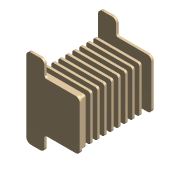
# Autodesk Inventor part: bobbin-2
Saved by Autodesk Inventor 2015 (Build 190159000, 159)
## iProperties
Created: 2014-10-07
Part Number: bobbin-2
Material: Polyethylene, Low Density
Document SubType Name: Modeling
Designer: Adam
Density: 0.894 g/cm^3
Appearance: Smooth - Off-White
Author: Adam
Autodesk Inventor part; units mm, degrees
ref_plane "Work Plane1" through (0, 0, 0.5) normal (0, 0, 1) x (1, 0, 0)
sketch "Sketch1" plane through (0, 0, 0.5) normal (0, 0, 1) x (1, 0, 0)
  line L0 (0, -12.7) -> (9.53, -12.7) construction
  line L1 (9.53, -4.565) -> (9.53, -12.7) construction
  line L2 (0, -4.565) -> (9.53, -4.565) construction
  line L3 (0, -4.565) -> (0, -12.7) construction
  line L4 (9.53, -22.23) -> (0, -22.23) construction
  line L5 (0, -22.23) -> (0, -30.365) construction
  line L6 (0, -30.365) -> (9.53, -30.365) construction
  line L7 (9.53, -22.23) -> (9.53, -30.365) construction
  line L8 (0, -22.23) -> (0, -12.7) construction
  line L9 (9.53, -12.7) -> (9.53, -22.23) construction
  line L10 (-0.5, -22.73) -> (10.03, -22.73)
  line L11 (10.03, -22.73) -> (10.03, -12.2)
  line L12 (10.03, -12.2) -> (-0.5, -12.2)
  line L13 (-0.5, -12.2) -> (-0.5, -22.73)
  line L14 (-0.5, -29.865) -> (10.03, -29.865)
  line L15 (10.03, -29.865) -> (10.03, -22.73)
  line L16 (10.03, -22.73) -> (-0.5, -22.73)
  line L17 (-0.5, -22.73) -> (-0.5, -29.865)
  line L18 (-0.5, -12.2) -> (10.03, -12.2)
  line L19 (10.03, -12.2) -> (10.03, -5.065)
  line L20 (10.03, -5.065) -> (-0.5, -5.065)
  line L21 (-0.5, -5.065) -> (-0.5, -12.2)
  line L22 (-0.5, -29.865) -> (-7.635, -29.865)
  line L23 (-7.635, -29.865) -> (-7.635, -5.065)
  line L24 (-7.635, -5.065) -> (-0.5, -5.065)
  line L25 (-0.5, -5.065) -> (-0.5, -29.865)
  line L26 (10.03, -29.865) -> (17.165, -29.865)
  line L27 (17.165, -29.865) -> (17.165, -5.065)
  line L28 (17.165, -5.065) -> (10.03, -5.065)
  line L29 (10.03, -5.065) -> (10.03, -29.865)
  point P0 (0, 0)
  dimension "d1" = 0.5
  dimension "d2" = 0.5
  dimension "d3" = 0.5
  dimension "d4" = 0.5
  dimension "d5" = 0.5
  dimension "d6" = 0.5
  dimension "d7" = 7.135
  dimension "d8" = 7.135
  dimension "d9" = 7.135
  constraints: 44 end point, 11 parallel, 5 horizontal, 5 perpendicular, 4 collinear, 1 vertical
  measures "d1" distance between parallel lines of L0 L12
  measures "d2" distance between parallel lines of L4 L10
  measures "d3" distance between parallel lines of L8 L13
  measures "d4" distance between parallel lines of L11 L9
  measures "d5" distance between parallel lines of L6 L14
  measures "d6" distance between parallel lines of L20 L2
  measures "d7" distance of L16.end L14.start
  measures "d8" distance between parallel lines of L23 L25
  measures "d9" distance between parallel lines of L11 L27
extrude "Extrusion1" add sketch "Sketch1" along normal blind 1.2 contours L17 L22 L23 L24 L21 L13 | L10 L15 L14 L17 | L11 L19 L28 L27 L26 L15 | L21 L20 L19 L12
sketch "Sketch2" plane through (0, 0, 1.7) normal (0, 0, 1) x (1, 0, 0)
  line L0 (-7.635, -29.865) -> (17.165, -29.865) construction
  line L1 (17.165, -29.865) -> (17.165, -5.065) construction
  line L2 (17.165, -5.065) -> (-7.635, -5.065) construction
  line L3 (-7.635, -5.065) -> (-7.635, -29.865) construction
  line L4 (-0.5, -22.73) -> (-0.5, -12.2) projected
  line L5 (-0.5, -12.2) -> (10.03, -12.2) projected
  line L6 (10.03, -12.2) -> (10.03, -22.73) projected
  line L7 (10.03, -22.73) -> (-0.5, -22.73) projected
  line L8 (-1.7, -23.93) -> (11.23, -23.93)
  line L9 (11.23, -23.93) -> (11.23, -11)
  line L10 (11.23, -11) -> (-1.7, -11)
  line L11 (-1.7, -11) -> (-1.7, -23.93)
  point P0 (0, 0)
  dimension "d12" = 1.2
  dimension "d13" = 1.2
  dimension "d14" = 1.2
  dimension "d15" = 1.2
  constraints: 8 end point, 2 parallel, 1 horizontal, 1 perpendicular
  measures "d12" distance between parallel lines of L4 L11
  measures "d13" distance between parallel lines of L8 L7
  measures "d14" distance between parallel lines of L10 L5
  measures "d15" distance between parallel lines of L6 L9
ref_plane "Work Plane2" through (0, -35.0828, 37.6) normal (0, 0, -1) x (1, 0, 0)
extrude "Extrusion2" add sketch "Sketch2" along normal up to surface (35.9 mm away)
sketch "Sketch3" plane through (-1.7, -23.93, 37.6) normal (0, 0, 1) x (1, 0, 0)
  line L0 (1.2, 11.73) -> (11.73, 11.73) construction
  line L1 (11.73, 11.73) -> (11.73, 1.2) construction
  line L2 (11.73, 1.2) -> (1.2, 1.2) construction
  line L3 (1.2, 1.2) -> (1.2, 11.73) construction
  line L4 (0, 12.93) -> (0, 0) construction
  line L5 (0, 0) -> (12.93, 0) construction
  line L6 (12.93, 0) -> (12.93, 12.93) construction
  line L7 (12.93, 12.93) -> (0, 12.93) construction
  line L8 (-5.935, -5.935) -> (18.865, -5.935)
  line L9 (18.865, -5.935) -> (18.865, 18.865)
  line L10 (18.865, 18.865) -> (-5.935, 18.865)
  line L11 (-5.935, 18.865) -> (-5.935, -5.935)
  line L12 (12.93, 0) -> (0, 0) construction
  line L13 (0, 0) -> (0, 12.93) construction
  line L14 (0, 12.93) -> (12.93, 12.93) construction
  line L15 (12.93, 12.93) -> (12.93, 0) construction
  line L16 (-5.935, -5.935) -> (18.865, -5.935) construction
  line L17 (18.865, -5.935) -> (18.865, 18.865) construction
  line L18 (18.865, 18.865) -> (-5.935, 18.865) construction
  line L19 (-5.935, 18.865) -> (-5.935, -5.935) construction
  line L20 (0, 0) -> (12.93, 0)
  line L21 (12.93, 0) -> (12.93, 12.93)
  line L22 (12.93, 12.93) -> (0, 12.93)
  line L23 (0, 12.93) -> (0, 0)
  point P0 (1.7, 23.93)
  constraints: 16 end point, 4 collinear, 4 parallel, 2 horizontal, 2 perpendicular
extrude "Extrusion3" add sketch "Sketch3" against normal blind 1.2
ref_plane "Work Plane3" through (-1.7, -23.93, 34.9) normal (0, 0, -1) x (-1, 0, 0)
sketch "Sketch4" plane through (-1.7, -23.93, 34.9) normal (0, 0, -1) x (-1, 0, 0)
  line L0 (5, 17.93) -> (-17.93, 17.93)
  line L1 (-17.93, 17.93) -> (-17.93, -5)
  line L2 (-17.93, -5) -> (5, -5)
  line L3 (5, -5) -> (5, 17.93)
  line L4 (0, 0) -> (0, 12.93) projected
  line L5 (-12.93, 0) -> (0, 0) projected
  line L6 (-12.93, 12.93) -> (-12.93, 0) projected
  line L7 (0, 12.93) -> (-12.93, 12.93) projected
  point P0 (-1.7, 23.93)
  dimension "d21" = 5
  dimension "d22" = 5
  dimension "d23" = 5
  dimension "d24" = 5
  constraints: 8 end point, 2 parallel, 1 horizontal, 1 perpendicular
  measures "d21" distance between parallel lines of L2 L5
  measures "d22" distance between parallel lines of L6 L1
  measures "d23" distance between parallel lines of L7 L0
  measures "d24" distance between parallel lines of L4 L3
extrude "Extrusion4" add sketch "Sketch4" along normal blind 1.2
fillet "Fillet1" radius 1 4 edges at (-6.7, -28.93, 34.3) (-6.7, -6, 34.3) (16.23, -28.93, 34.3) (16.23, -6, 34.3)
pattern_linear "Rectangular Pattern1" count 9 spacing 3.5 along (0, 0, -1) of "Extrusion4", "Fillet1"
fillet "Fillet2" radius 2 8 edges at (-7.635, -29.865, 37) (17.165, -29.865, 37) (17.165, -5.065, 37) (-7.635, -5.065, 37) (-7.635, -5.065, 1.1) (-7.635, -29.865, 1.1) (17.165, -29.865, 1.1) (17.165, -5.065, 1.1)
fillet "Fillet2" radius 1.5 4 edges at (11.23, -11, 3.7) (11.23, -23.93, 3.7) (-1.7, -11, 3.7) (-1.7, -23.93, 3.7)
fillet "Fillet2" radius 1 4 edges at (-0.5, -12.2, 19.05) (-0.5, -22.73, 19.05) (10.03, -22.73, 19.05) (10.03, -12.2, 19.05)
sketch "Sketch5" plane through (-5.635, -29.865, 37.6) normal (0, 0, 1) x (1, 0, 0)
  arc A0 (0, 24.8) -> (-2, 22.8) centre (0, 22.8) ccw construction
  line L0 (-2, 22.8) -> (-2, 2) construction
  arc A1 (-2, 2) -> (0, 0) centre (0, 2) ccw construction
  line L1 (0, 0) -> (20.8, 0) construction
  arc A2 (20.8, 0) -> (22.8, 2) centre (20.8, 2) ccw construction
  line L2 (22.8, 2) -> (22.8, 22.8) construction
  arc A3 (22.8, 22.8) -> (20.8, 24.8) centre (20.8, 22.8) ccw construction
  line L3 (20.8, 24.8) -> (0, 24.8) construction
  line L4 (6.135, 17.665) -> (14.665, 17.665) construction
  line L5 (15.665, 16.665) -> (15.665, 8.135) construction
  line L6 (14.665, 7.135) -> (6.135, 7.135) construction
  line L7 (5.135, 8.135) -> (5.135, 16.665) construction
  arc A4 (0, 24.8) -> (-2, 22.8) centre (0, 22.8) ccw projected
  line L8 (0, 24.8) -> (20.8, 24.8) projected
  arc A5 (22.8, 22.8) -> (20.8, 24.8) centre (20.8, 22.8) ccw projected
  line L9 (22.8, 22.8) -> (22.8, 2) projected
  arc A6 (20.8, 0) -> (22.8, 2) centre (20.8, 2) ccw projected
  line L10 (20.8, 0) -> (0, 0) projected
  arc A7 (-2, 2) -> (0, 0) centre (0, 2) ccw projected
  line L11 (-2, 2) -> (-2, 22.8) projected
  line L12 (16.865, 17.365) -> (16.865, 7.435) projected
  line L13 (5.435, 18.865) -> (15.365, 18.865) projected
  line L14 (3.935, 7.435) -> (3.935, 17.365) projected
  line L15 (15.365, 5.935) -> (5.435, 5.935) projected
  line L16 (3.435, 4.435) -> (17.365, 4.435)
  line L17 (18.365, 5.435) -> (18.365, 19.365)
  line L18 (17.365, 20.365) -> (3.435, 20.365)
  line L19 (2.435, 19.365) -> (2.435, 5.435)
  arc A8 (2.435, 5.435) -> (3.435, 4.435) centre (3.435, 5.435) ccw
  arc A9 (17.365, 4.435) -> (18.365, 5.435) centre (17.365, 5.435) ccw
  arc A10 (18.365, 19.365) -> (17.365, 20.365) centre (17.365, 19.365) ccw
  arc A11 (3.435, 20.365) -> (2.435, 19.365) centre (3.435, 19.365) ccw
  arc A12 (15.665, 16.665) -> (14.665, 17.665) centre (14.665, 16.665) ccw projected
  arc A13 (14.665, 7.135) -> (15.665, 8.135) centre (14.665, 8.135) ccw projected
  arc A14 (5.135, 8.135) -> (6.135, 7.135) centre (6.135, 8.135) ccw projected
  arc A15 (6.135, 17.665) -> (5.135, 16.665) centre (6.135, 16.665) ccw projected
  arc A16 (15.365, 5.935) -> (16.865, 7.435) centre (15.365, 7.435) ccw projected
  arc A17 (16.865, 17.365) -> (15.365, 18.865) centre (15.365, 17.365) ccw projected
  arc A18 (5.435, 18.865) -> (3.935, 17.365) centre (5.435, 17.365) ccw projected
  arc A19 (3.935, 7.435) -> (5.435, 5.935) centre (5.435, 7.435) ccw projected
  point P0 (5.635, 29.865)
  dimension "d32" = 1.5
  dimension "d33" = 1.5
  dimension "d34" = 1.5
  dimension "d35" = 1.5
  dimension "d36" = 1
  constraints: 8 end point, 8 point on circle, 8 tangent, 4 centre point, 3 equal radius, 2 parallel, 1 horizontal, 1 perpendicular
  measures "d32" distance between parallel lines of L18 L13
  measures "d33" distance between parallel lines of L14 L19
  measures "d34" distance between parallel lines of L16 L15
  measures "d35" distance between parallel lines of L17 L12
  measures "d36" radius of A8
extrude "Extrusion5" add sketch "Sketch5" against normal up to surface (30.7 mm away) contours A8 L19 A11 L18 A10 L17 A9 L16
sketch "Sketch6" plane through (-6.7, -27.93, 10.4) normal (-1, 0, 0) x (0, 0, 1)
  line L0 (5.8, 20.93) -> (7, 20.93) construction
  line L1 (5.8, 0) -> (5.8, 20.93) construction
  line L2 (7, 0) -> (5.8, 0) construction
  line L3 (7, 0) -> (7, 20.93) construction
  line L4 (9.3, 20.93) -> (10.5, 20.93) construction
  line L5 (9.3, 0) -> (9.3, 20.93) construction
  line L6 (10.5, 0) -> (9.3, 0) construction
  line L7 (10.5, 0) -> (10.5, 20.93) construction
  line L8 (12.8, 20.93) -> (14, 20.93) construction
  line L9 (12.8, 0) -> (12.8, 20.93) construction
  line L10 (14, 0) -> (12.8, 0) construction
  line L11 (14, 0) -> (14, 20.93) construction
  line L12 (16.3, 20.93) -> (17.5, 20.93) construction
  line L13 (16.3, 0) -> (16.3, 20.93) construction
  line L14 (17.5, 0) -> (16.3, 0) construction
  line L15 (17.5, 0) -> (17.5, 20.93) construction
  line L16 (19.8, 20.93) -> (21, 20.93) construction
  line L17 (19.8, 0) -> (19.8, 20.93) construction
  line L18 (21, 0) -> (19.8, 0) construction
  line L19 (21, 0) -> (21, 20.93) construction
  line L20 (23.3, 20.93) -> (24.5, 20.93) construction
  line L21 (23.3, 0) -> (23.3, 20.93) construction
  line L22 (24.5, 0) -> (23.3, 0) construction
  line L23 (24.5, 0) -> (24.5, 20.93) construction
  line L24 (2.3, 20.93) -> (3.5, 20.93) construction
  line L25 (2.3, 0) -> (2.3, 20.93) construction
  line L26 (3.5, 0) -> (2.3, 0) construction
  line L27 (3.5, 0) -> (3.5, 20.93) construction
  line L28 (2.3, 0) -> (2.3, 20.93)
  line L29 (2.3, 11.965) -> (3.5, 11.965)
  line L30 (3.5, 11.965) -> (3.5, 8.965)
  line L31 (3.5, 8.965) -> (2.3, 8.965)
  line L32 (2.3, 8.965) -> (2.3, 11.965)
  line L33 (5.8, 0) -> (5.8, 20.93)
  line L34 (7, 3.5) -> (7, 17.43)
  line L35 (5.8, 11.965) -> (7, 11.965)
  line L36 (7, 11.965) -> (7, 8.965)
  line L37 (7, 8.965) -> (5.8, 8.965)
  line L38 (5.8, 8.965) -> (5.8, 11.965)
  line L39 (9.3, 17.43) -> (9.3, 3.5)
  line L40 (10.5, 0) -> (10.5, 20.93)
  line L41 (9.3, 11.965) -> (10.5, 11.965)
  line L42 (10.5, 11.965) -> (10.5, 8.965)
  line L43 (10.5, 8.965) -> (9.3, 8.965)
  line L44 (9.3, 8.965) -> (9.3, 11.965)
  line L45 (12.8, 17.43) -> (12.8, 3.5)
  line L46 (12.8, 11.965) -> (14, 11.965)
  line L47 (14, 11.965) -> (14, 8.965)
  line L48 (14, 8.965) -> (12.8, 8.965)
  line L49 (12.8, 8.965) -> (12.8, 11.965)
  line L50 (17.5, 17.43) -> (17.5, 3.5)
  line L51 (16.3, 11.965) -> (17.5, 11.965)
  line L52 (17.5, 11.965) -> (17.5, 8.965)
  line L53 (17.5, 8.965) -> (16.3, 8.965)
  line L54 (16.3, 8.965) -> (16.3, 11.965)
  line L55 (21, 17.43) -> (21, 3.5)
  line L56 (19.8, 11.965) -> (21, 11.965)
  line L57 (21, 11.965) -> (21, 8.965)
  line L58 (21, 8.965) -> (19.8, 8.965)
  line L59 (19.8, 8.965) -> (19.8, 11.965)
  line L60 (23.3, 11.965) -> (24.5, 11.965)
  line L61 (24.5, 11.965) -> (24.5, 8.965)
  line L62 (24.5, 8.965) -> (23.3, 8.965)
  line L63 (23.3, 8.965) -> (23.3, 11.965)
  line L64 (2.3, 10.465) -> (24.5, 10.465) construction
  line L65 (24.5, 20.93) -> (24.5, 0) construction
  line L66 (0, 3.5) -> (0, 17.43)
  line L67 (0, 8.965) -> (-1.2, 8.965)
  line L68 (-1.2, 8.965) -> (-1.2, 11.965)
  line L69 (-1.2, 11.965) -> (0, 11.965)
  line L70 (0, 11.965) -> (0, 8.965)
  line L71 (-1.2, 0) -> (-1.2, 20.93)
  line L72 (-3.5, 14.73) -> (-3.5, 6.2)
  line L73 (-4.7, 9.465) -> (-3.5, 9.465)
  line L74 (-3.5, 9.465) -> (-3.5, 11.465)
  line L75 (-3.5, 11.465) -> (-4.7, 11.465)
  line L76 (-4.7, 11.465) -> (-4.7, 9.465)
  line L77 (-4.7, 0) -> (-4.7, 20.93)
  point P0 (-10.4, 27.93)
extrude "Extrusion6" cut sketch "Sketch6" against normal up to surface (3.5 mm away) contours L28 L29 L30 L31 | L33 L35 L34 L37 | L41 L40 L43 L39 | L46 L47 L48 L45 | L50 L53 L54 L51 | L55 L58 L59 L56 | L67 L68 L69 L66 | L72 L73 L76 L75
sketch "Sketch7" plane through (0, 0, 0.5) normal (0, 0, -1) x (-1, 0, 0)
  line L0 (-10.03, -13.2) -> (-10.03, -21.73) projected
  line L1 (-0.5, -12.2) -> (-9.03, -12.2) projected
  line L2 (0.5, -21.73) -> (0.5, -13.2) projected
  line L3 (-9.03, -22.73) -> (-0.5, -22.73) projected
  arc A0 (-15.165, -5.065) -> (-17.165, -7.065) centre (-15.165, -7.065) ccw projected
  line L4 (-17.165, -27.865) -> (-17.165, -7.065) projected
  arc A1 (-17.165, -27.865) -> (-15.165, -29.865) centre (-15.165, -27.865) ccw projected
  line L5 (5.635, -29.865) -> (-15.165, -29.865) projected
  arc A2 (5.635, -29.865) -> (7.635, -27.865) centre (5.635, -27.865) ccw projected
  line L6 (7.635, -7.065) -> (7.635, -27.865) projected
  arc A3 (7.635, -7.065) -> (5.635, -5.065) centre (5.635, -7.065) ccw projected
  line L7 (-15.165, -5.065) -> (5.635, -5.065) projected
  line L8 (-9.865, 3.035) -> (7.135, 3.035) projected
  line L9 (7.135, -37.965) -> (-9.865, -37.965) projected
  arc A4 (7.135, -37.965) -> (10.135, -34.965) centre (7.135, -34.965) ccw projected
  arc A5 (10.135, 0.035) -> (7.135, 3.035) centre (7.135, 0.035) ccw projected
  line L10 (5.635, -29.865) -> (-15.165, -29.865) projected
  line L11 (0.5, -29.865) -> (0.5, -37.465)
  line L12 (0.5, -37.465) -> (7.135, -37.465)
  arc A6 (7.135, -37.465) -> (9.635, -34.965) centre (7.135, -34.965) ccw
  line L13 (9.635, -34.965) -> (9.635, 0.035)
  arc A7 (9.635, 0.035) -> (7.135, 2.535) centre (7.135, 0.035) ccw
  line L14 (-15.165, -5.065) -> (5.635, -5.065) construction
  line L15 (0.5, -5.065) -> (0.5, 2.535)
  line L16 (0.5, 2.535) -> (7.135, 2.535)
  line L17 (0, 0) -> (0, -34.93) construction
  line L18 (0.5, -29.865) -> (5.635, -29.865)
  arc A8 (5.635, -29.865) -> (7.635, -27.865) centre (5.635, -27.865) ccw projected
  arc A9 (5.635, -29.865) -> (7.635, -27.865) centre (5.635, -27.865) ccw
  arc A10 (7.635, -7.065) -> (5.635, -5.065) centre (5.635, -7.065) ccw
  line L19 (7.635, -27.865) -> (7.635, -7.065)
  line L20 (5.635, -5.065) -> (0.5, -5.065)
  line L21 (-9.53, -34.93) -> (0, -34.93) construction
  line L22 (-9.53, 0) -> (0, 0) construction
  line L23 (-9.53, 0) -> (-9.53, -34.93) construction
  line L24 (0.5, -37.465) -> (-14.03, -37.465)
  line L25 (-14.03, -37.465) -> (-14.03, -35.43)
  line L26 (-10.03, -35.43) -> (0.5, -35.43)
  line L27 (0.5, -35.43) -> (0.5, -37.465)
  line L28 (0.5, 2.535) -> (-10.03, 2.535)
  line L29 (-10.03, 0.5) -> (0.5, 0.5)
  line L30 (0.5, 0.5) -> (0.5, 2.535)
  line L31 (-10.03, -35.43) -> (-10.03, -29.865)
  line L32 (-10.03, -29.865) -> (-14.03, -29.865)
  line L33 (-14.03, -29.865) -> (-14.03, -35.43)
  line L34 (-14.03, -5.065) -> (-10.03, -5.065)
  line L35 (-10.03, -5.065) -> (-10.03, 0.5)
  line L36 (-10.03, 2.535) -> (-14.03, 2.535)
  line L37 (-14.03, 2.535) -> (-14.03, -5.065)
  arc A11 (-10.03, -21.73) -> (-9.03, -22.73) centre (-9.03, -21.73) ccw projected
  arc A12 (-9.03, -12.2) -> (-10.03, -13.2) centre (-9.03, -13.2) ccw projected
  arc A13 (0.5, -13.2) -> (-0.5, -12.2) centre (-0.5, -13.2) ccw projected
  arc A14 (-0.5, -22.73) -> (0.5, -21.73) centre (-0.5, -21.73) ccw projected
  dimension "d46" = 0.5
  dimension "d48" = 0.5
  dimension "d52" = 0.5
  dimension "d53" = 0.5
  dimension "d54" = 0.5
  dimension "d55" = 4
  constraints: 44 end point, 8 point on circle, 6 parallel, 6 tangent, 5 perpendicular, 5 point on line, 4 centre point, 4 coincident, 4 collinear, 4 horizontal, 3 vertical
  measures "d46" distance between parallel lines of L8 L16
  measures "d48" distance between parallel lines of L17 L11
  measures "d52" distance between parallel lines of L21 L26
  measures "d53" distance between parallel lines of L22 L29
  measures "d54" distance between parallel lines of L23 L35
  measures "d55" distance between parallel lines of L31 L33
extrude "Extrusion7" add sketch "Sketch7" against normal up to surface (1.2 mm away) contours L15 L16 A7 L13 A6 L12 L11 L5 A2 L6 A3 L7
ref_plane "Work Plane5" through (0, 0, 19.05) normal (0, 0, -1) x (-1, 0, 0)
mirror "Mirror2" about plane through (0, 0, 19.05) normal (0, 0, -1) of "Extrusion7"
fillet "Fillet6" radius 1 4 edges at (-0.5, -29.865, 1.1) (-0.5, -5.065, 1.1) (-0.5, -5.065, 37) (-0.5, -29.865, 37)
ref_plane "Work Plane6" through (0, 0, 0.25) normal (0, 0, -1) x (-1, 0, 0)
ref_plane "Work Plane7" through (0, 0, 1.1) normal (0, 0, -1) x (-1, 0, 0)
ref_plane "Work Plane8" through (-1.7, -23.93, 36.15) normal (0, 0, -1) x (-1, 0, 0)
ref_plane "Work Plane9" through (17.165, -27.865, 37) normal (0, 0, 1) x (1, 0, 0)
sketch "Sketch8" plane through (0, 0, 0.5) normal (0, 0, -1) x (-1, 0, 0)
  line L0 (0.5, -37.465) -> (7.135, -37.465) projected
  arc A0 (7.135, -37.465) -> (9.635, -34.965) centre (7.135, -34.965) ccw projected
  line L1 (9.635, -34.965) -> (9.635, 0.035) projected
  arc A1 (9.635, 0.035) -> (7.135, 2.535) centre (7.135, 0.035) ccw projected
  line L2 (7.135, 2.535) -> (0.5, 2.535) projected
  arc A2 (-15.165, -5.065) -> (-17.165, -7.065) centre (-15.165, -7.065) ccw projected
  line L3 (-17.165, -27.865) -> (-17.165, -7.065) projected
  arc A3 (-17.165, -27.865) -> (-15.165, -29.865) centre (-15.165, -27.865) ccw projected
  arc A4 (0.5, -30.865) -> (-0.5, -29.865) centre (-0.5, -30.865) ccw projected
  line L4 (0.5, -30.865) -> (0.5, -37.465) projected
  line L5 (-0.5, -29.865) -> (-15.165, -29.865) projected
  line L6 (0.5, 2.535) -> (0.5, -4.065) projected
  arc A5 (-0.5, -5.065) -> (0.5, -4.065) centre (-0.5, -4.065) ccw projected
  line L7 (-15.165, -5.065) -> (-0.5, -5.065) projected
  arc A6 (-10.03, -21.73) -> (-9.03, -22.73) centre (-9.03, -21.73) ccw projected
  line L8 (-10.03, -13.2) -> (-10.03, -21.73) projected
  arc A7 (-9.03, -12.2) -> (-10.03, -13.2) centre (-9.03, -13.2) ccw projected
  line L9 (-0.5, -12.2) -> (-9.03, -12.2) projected
  arc A8 (0.5, -13.2) -> (-0.5, -12.2) centre (-0.5, -13.2) ccw projected
  line L10 (0.5, -21.73) -> (0.5, -13.2) projected
  arc A9 (-0.5, -22.73) -> (0.5, -21.73) centre (-0.5, -21.73) ccw projected
  line L11 (-9.03, -22.73) -> (-0.5, -22.73) projected
  line L12 (-0.5, -35.43) -> (-9.03, -35.43) projected
  circle A10 centre (-4.765, -35.43) radius 0.75
  line L13 (-9.03, 0.5) -> (-0.5, 0.5) projected
  circle A11 centre (-4.765, 0.5) radius 0.75
  point P0 (0, 0)
  dimension "d64" = 1.5
  constraints: 2 centre point, 2 midpoint, 1 equal radius
  measures "d64" diameter of A10
extrude "Extrusion8" [suppressed]
fillet "Fillet7" [suppressed]
sketch "Sketch10" plane through (-1.7, -23.93, 34.9) normal (0, 0, 1) x (1, 0, 0)
  line L0 (-1.5, -0.5) -> (-1.5, 13.43) projected
  arc A0 (-0.5, 14.43) -> (-1.5, 13.43) centre (-0.5, 13.43) ccw projected
  line L1 (-0.5, 14.43) -> (13.43, 14.43) projected
  arc A1 (14.43, 13.43) -> (13.43, 14.43) centre (13.43, 13.43) ccw projected
  line L2 (14.43, 13.43) -> (14.43, -0.5) projected
  arc A2 (13.43, -1.5) -> (14.43, -0.5) centre (13.43, -0.5) ccw projected
  line L3 (13.43, -1.5) -> (-0.5, -1.5) projected
  arc A3 (-1.5, -0.5) -> (-0.5, -1.5) centre (-0.5, -0.5) ccw projected
  arc A4 (17.93, 16.93) -> (16.93, 17.93) centre (16.93, 16.93) ccw projected
  line L4 (-4, 17.93) -> (16.93, 17.93) projected
  arc A5 (-4, 17.93) -> (-5, 16.93) centre (-4, 16.93) ccw projected
  line L5 (-5, -4) -> (-5, 16.93) projected
  arc A6 (-5, -4) -> (-4, -5) centre (-4, -4) ccw projected
  line L6 (16.93, -5) -> (-4, -5) projected
  arc A7 (16.93, -5) -> (17.93, -4) centre (16.93, -4) ccw projected
  line L7 (17.93, 16.93) -> (17.93, -4) projected
  point P0 (1.7, 23.93)
extrude "Extrusion9" add sketch "Sketch10" along normal up to next
fillet "Fillet8" radius 2 4 edges at (-0.5, 2.535, 1.1) (-0.5, -37.465, 1.1) (-0.5, 2.535, 37) (-0.5, -37.465, 37)
equation "\"d1\" = d0"
equation "\"d2\" = d1"
equation "\"d3\" = d1"
equation "\"d4\" = d1"
equation "\"d8\" = d7"
equation "\"d9\" = d7"
equation "\"d12\" = d10"
equation "\"d13\" = d10"
equation "\"d14\" = d10"
equation "\"d15\" = d10"
equation "\"d18\" = d10"
equation "\"d22\" = d21"
equation "\"d23\" = d21"
equation "\"d24\" = d21"
equation "\"d25\" = d10"
equation "\"d33\" = d32"
equation "\"d34\" = d32"
equation "\"d35\" = d32"
equation "\"d48\" = d46"
equation "\"d52\" = d46"
equation "\"d53\" = d46"
equation "\"d54\" = d46"
equation "\"d0\" = 0.5"
equation "\"d10\" = 1.2"
body "Solid1"
